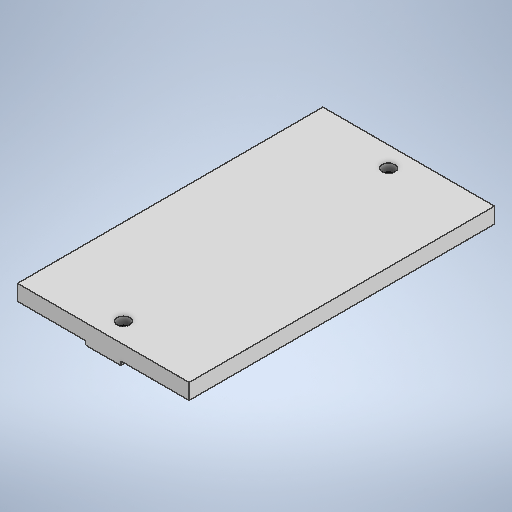
# Autodesk Inventor part: plathomeusbhub
Saved by Autodesk Inventor 2025 (Build 290162000, 162)
## iProperties
Created: 2025-10-23
Part Number: plathomeusbhub
Material: 一般
Document SubType Name: Modeling
Designer: sooo1
Density: 1 g/cm^3
Appearance: 既定
Author: sooo1
Autodesk Inventor part; units mm, degrees
ref_plane "YZ Plane" through (0, 0, 0) normal (1, 0, 0) x (0, 1, 0)
ref_plane "XZ Plane" through (0, 0, 0) normal (0, 1, 0) x (-1, 0, 0)
ref_plane "XY Plane" through (0, 0, 0) normal (0, 0, 1) x (1, 0, 0)
sketch "スケッチ1" plane through (0, 0, 0) normal (0, 1, 0) x (-1, 0, 0)
  line L0 (22, 39.15) -> (-22, 39.15)
  line L1 (-22, 39.15) -> (-22, -39.15)
  line L2 (-22, -39.15) -> (22, -39.15)
  line L3 (22, -39.15) -> (22, 39.15)
  line L4 (22, 39.15) -> (-22, -39.15) construction
  line L5 (-22, 39.15) -> (22, -39.15) construction
  line L6 (0, -54.81) -> (0, 54.81) construction
  line L7 (30.8, 0) -> (-30.8, 0) construction
  circle A0 centre (0, 34) radius 1.65
  circle A1 centre (0, -34) radius 1.65
  circle A2 centre (0, 17.5) radius 3.075
  circle A3 centre (0, -17.5) radius 3.075
  circle A4 centre (0, 34) radius 3
  circle A5 centre (0, -34) radius 3
  line L8 (-4.5, 39.15) -> (-4.5, -39.15)
  line L9 (4.5, 39.15) -> (4.5, -39.15)
  point P0 (0, 0)
  dimension "d0" = 3.3
  dimension "d2" = 44
  dimension "d3" = 78.3
  dimension "d4" = 68
  dimension "d7" = 6.15
  dimension "d8" = 35
  dimension "d9" = 6
  dimension "d14" = 17.5
  constraints: 16 end point, 6 centre point, 5 symmetric about line, 4 point on line, 2 midpoint, 2 parallel, 2 perpendicular, 1 coincident, 1 horizontal, 3 other
  measures "d0" diameter of A0
  measures "d2" distance of L0.start L0.end
  measures "d3" distance of L2.end L0.start
  measures "d4" diameter of A0.centre L7
  measures "d7" diameter of A2
  measures "d8" diameter of A2.centre L7
  measures "d9" diameter of A4
  measures "d14" distance between parallel lines of L1 L8
extrude "押し出し1" add sketch "スケッチ1" along normal blind 5 contours L3 L2 L9 L0 | L9 L2 L8 L0 | L8 L2 L1 L0 | A2 | A3 | A4 | A5
extrude "押し出し2" cut sketch "スケッチ1" along normal blind 3 contours A2 | A3
extrude "押し出し3" cut sketch "スケッチ1" along normal blind 3 contours A0 | A1 | A4 | A5
extrude "押し出し4" cut sketch "スケッチ1" along normal blind 1 contours L3 L2 L9 L0 | L8 L2 L1 L0
